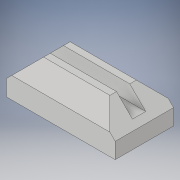
# Autodesk Inventor part: Block
Saved by Autodesk Inventor 2019 (Build 230136000, 136)
## iProperties
Created: 2018-11-05
Part Number: Block
Material: Generic
Document SubType Name: Modeling
Designer: 2003189
Density: 1 g/cm^3
Appearance: Default
Author: 2003189
Autodesk Inventor part; units mm, degrees
ref_plane "YZ Plane" through (0, 0, 0) normal (1, 0, 0) x (0, 1, 0)
ref_plane "XZ Plane" through (0, 0, 0) normal (0, 1, 0) x (-1, 0, 0)
ref_plane "XY Plane" through (0, 0, 0) normal (0, 0, 1) x (1, 0, 0)
sketch "Sketch1" plane through (0, 0, 0) normal (0, 1, 0) x (-1, 0, 0)
  line L0 (0, 0) -> (130.175, 0)
  line L1 (130.175, 0) -> (130.175, -69.85)
  line L2 (130.175, -69.85) -> (0, -69.85)
  line L3 (0, -69.85) -> (0, 0)
  dimension "d0" = 130.175
  dimension "d1" = 69.85
  constraints: 8 end point, 2 parallel, 1 horizontal, 1 perpendicular
  measures "d0" distance of L1.end L2.end
  measures "d1" distance of L0.end L1.end
extrude "Extrusion1" add sketch "Sketch1" along normal blind 44.45
sketch "Sketch2" plane through (0, 44.45, 0) normal (0, 1, 0) x (1, 0, 0)
  line L0 (0, 0) -> (0, 69.85) projected
  line L1 (0, 0) -> (0, 34.925)
  line L2 (0, 34.925) -> (-130.175, 34.925)
  line L3 (-130.175, 69.85) -> (-130.175, 0) projected
  line L4 (-130.175, 34.925) -> (0, 34.925)
  line L5 (0, 34.925) -> (0, 26.9875)
  line L6 (0, 26.9875) -> (-130.175, 26.9875)
  line L7 (-130.175, 26.9875) -> (-130.175, 34.925)
  line L8 (0, 26.9875) -> (-25.3296, 26.9875)
  line L9 (-25.3296, 26.9875) -> (-25.3296, 42.8625)
  line L10 (-25.3296, 42.8625) -> (0, 42.8625)
  line L11 (0, 42.8625) -> (0, 26.9875)
  line L12 (0, 26.9875) -> (-130.175, 26.9875)
  line L13 (-130.175, 26.9875) -> (-130.175, 42.8625)
  line L14 (-130.175, 42.8625) -> (0, 42.8625)
  line L15 (0, 42.8625) -> (0, 26.9875)
  dimension "d4" = 7.9375
  dimension "d5" = 15.875
  constraints: 28 end point, 6 parallel, 3 horizontal, 3 perpendicular, 2 midpoint, 2 point on line
  measures "d4" distance of L4.end L5.end
  measures "d5" distance of L8.end L9.end
extrude "Extrusion2" cut sketch "Sketch2" against normal blind 19.05
chamfer "Chamfer1" distance 25.4 angle 45 2 edges at (0, 44.45, -13.4937) (-130.175, 44.45, -13.4938)
chamfer "Chamfer2" distance 19.05 angle 45 2 edges at (-65.0875, 44.45, 0) (-65.0875, 44.45, -69.85)
body "Solid1"
